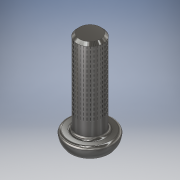
# Autodesk Inventor part: Parafuso m5 16mm
Saved by Autodesk Inventor 2019.4 (Build 234330000, 330)
## iProperties
Created: 2021-05-17
Part Number: Parafuso m5 16mm
Material: Aço, carbono
Document SubType Name: Modeling
Designer: Lattes
Density: 7.85 g/cm^3
Appearance: Aço - Polido
Author: Lattes
Autodesk Inventor part; units mm, degrees
ref_plane "YZ Plane" through (0, 0, 0) normal (1, 0, 0) x (0, 1, 0)
ref_plane "XZ Plane" through (0, 0, 0) normal (0, 1, 0) x (-1, 0, 0)
ref_plane "XY Plane" through (0, 0, 0) normal (0, 0, 1) x (1, 0, 0)
sketch "Esboço1" plane through (0, 0, 0) normal (0, 1, 0) x (-1, 0, 0)
  circle A0 centre (0, 0) radius 4.375
  dimension "d0" = 8.75
  constraints: 1 centre point, 1 coincident
  measures "d0" diameter of A0
extrude "Extrusão1" add sketch "Esboço1" along normal blind 3
sketch "Esboço2" plane through (0, 3, 0) normal (0, 1, 0) x (1, 0, 0)
  circle A0 centre (0, 0) radius 2.5
  dimension "d3" = 5
  constraints: 1 centre point, 1 coincident
  measures "d3" diameter of A0
extrude "Extrusão2" add sketch "Esboço2" along normal blind 16
thread "Rosca1" size "M5x0.8" class "6g" standard "ANSI Metric M Profile" length 13
chamfer "Chanfro1" distance 0.5 angle 45 1 edges at (-2.5, 19, 0)
fillet "Arredondamento1" radius 0.5 2 edges at (-2.5, 3, 0) (4.375, 3, 0)
sketch "Esboço3" plane through (0, 0, 0) normal (0, -1, 0) x (1, 0, 0)
  point P0 (0, 0)
sketch "Esboço4" plane through (0, 0, 0) normal (1, 0, 0) x (0, 1, 0)
  line L0 (2.55, -1.375) -> (0, -2.375)
  line L1 (0, 0) -> (2.55, 0)
  line L2 (2.55, 0) -> (2.55, -1.375)
  line L3 (0, 0) -> (0, -2.375)
  point P0 (0, -4.375)
  dimension "d12" = 2
  constraints: 8 end point, 1 parallel, 1 perpendicular
  measures "d12" distance of point (0, -4.375) L0.end
extrude "Extrusão3" cut sketch "Esboço4" along normal mid plane 1
pattern_circular "Padrão circular1" count 4 over 360 about axis through (0, -10, 0) along (0, 1, 0) of "Extrusão3"
fillet "Arredondamento2" radius 0.5 4 edges at (0.5, 1.275, -0.5) (0.5, 1.275, 0.5) (-0.5, 1.275, 0.5) (-0.5, 1.275, -0.5)
fillet "Arredondamento3" radius 0.15 38 edges at (2.375, 0, 0) (1.875, 1.275, 0.5) (1.875, 1.275, -0.5) (1.375, 2.55, 0) (0, 0, 2.375) (0.5, 1.275, 1.875) (0, 0, -2.375) (0, 2.55, -1.375) (-1.375, 2.55, 0) (0, 2.55, 1.375) (-0.5, 1.275, 1.875) (-1.875, 1.275, -0.5) (-0.5, 1.275, -1.875) (0.5, 1.275, -1.875) (-1.875, 1.275, 0.5) (-2.375, 0, 0) (-0.5, 0, -1.6875) (-1.6875, 0, -0.5) (-0.6464, 0, -0.6464) (-0.6464, 0, 0.6464) (-0.5, 0, 1.6875) (-1.6875, 0, 0.5) (0.6464, 0, 0.6464) (1.6875, 0, 0.5) (0.5, 0, 1.6875) (0.5, 0, -1.6875) (0.6464, 0, -0.6464) (1.1875, 2.55, 0.5) (0.5, 2.55, 1.1875) (0.6464, 2.55, 0.6464) (0.5, 2.55, -1.1875) (-1.1875, 2.55, -0.5) (0.6464, 2.55, -0.6464) (-0.6464, 2.55, 0.6464) (-0.5, 2.55, 1.1875) (-1.1875, 2.55, 0.5) (-0.5, 2.55, -1.1875) (-0.6464, 2.55, -0.6464)
sketch "Esboço5" plane through (0, 0, 0) normal (0, 0, 1) x (1, 0, 0)
  line L0 (0, 0) -> (0, 3.8786)
  line L1 (0, 3.8786) -> (0, -1.6488)
  arc A0 (0, 0) -> (3.4564, 0.5587) centre (0.0922, 10.4009) ccw
  arc A1 (3.6675, 0.6986) -> (4.375, 2.5) centre (1.5918, 2.5534) ccw
  arc A2 (3.4564, 0.5587) -> (3.6675, 0.6986) centre (3.2947, 1.0318) ccw
  line L2 (4.375, 2.5) -> (4.375, 0)
  line L3 (4.375, 0) -> (0, 0)
  line L4 (0.35, 0) -> (-0.35, 0) projected
  line L5 (-4.375, 0) -> (4.375, 0) projected
  line L6 (0.1845, 0) -> (4.375, 0)
  line L7 (4.375, 0) -> (4.375, 2.5)
  dimension "d25" = 0.5
  constraints: 12 end point, 7 point on circle, 3 centre point, 2 point on line, 2 tangent, 1 horizontal, 1 perpendicular, 1 vertical
  measures "d25" radius of A2
revolve "Revolução1" cut sketch "Esboço5" angle 360 about axis through (0, 3.8786, 0) along (0, -1, 0)
